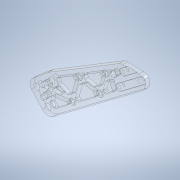
# Autodesk Inventor part: アーム アーム先端根本ポリカパーツ
Saved by Autodesk Inventor 2020.2 (Build 242310000, 310)
## iProperties
Created: 2020-05-02
Part Number: アーム アーム先端根本ポリカパーツ
Material: ポリカーボネート、クリア
Document SubType Name: Modeling
Designer: mozar
Density: 1.2 g/cm^3
Appearance: ポリカーボネート - クリア
Mass: 15.4398 g
Surface Area: 103.612 cm^2
Volume: 12.8665 cm^3
Author: mozar
Autodesk Inventor part; units mm, degrees
(part 1 of 2)
ref_plane "YZ Plane" through (0, 0, 0) normal (1, 0, 0) x (0, 1, 0)
ref_plane "XZ Plane" through (0, 0, 0) normal (0, 1, 0) x (-1, 0, 0)
ref_plane "XY Plane" through (0, 0, 0) normal (0, 0, 1) x (1, 0, 0)
sketch "スケッチ1" plane through (0, 0, 0) normal (0, 0, 1) x (1, 0, 0)
  circle A0 centre (-129.11052, 24.304119) radius 1.5
  circle A1 centre (-99.752673, 43.359743) radius 1.5
  circle A2 centre (-45.703772, 62.415368) radius 1.5
  circle A3 centre (-41.036979, 81.470992) radius 1.5
  circle A4 centre (-70.394826, 62.415368) radius 1.5
  circle A5 centre (-73.694174, 41.402576) radius 1.5
  circle A6 centre (-101.684575, 20.389785) radius 1.5
  circle A7 centre (-147.951739, 7.872185) radius 1.5
  line L0 (-23.449069, 99.142406) -> (-7.448842, 98.649717)
  arc A8 (-3.447491, 86.009971) -> (-7.448842, 98.649717) centre (-7.665058, 91.628045) ccw
  line L1 (-3.447491, 86.009971) -> (-131.660668, -10.24148)
  arc A9 (-141.440781, -10.106867) -> (-131.660668, -10.24148) centre (-136.463592, -3.843674) ccw
  line L2 (-141.440781, -10.106867) -> (-154.18878, 0.023621)
  arc A10 (-153.409815, 16.281111) -> (-154.18878, 0.023621) centre (-147.951739, 7.872185) ccw
  line L3 (-153.409815, 16.281111) -> (-27.490021, 98.013273)
  arc A11 (-23.449069, 99.142406) -> (-27.490021, 98.013273) centre (-23.665285, 92.120734) ccw
  circle A12 centre (-136.463592, -3.843674) radius 1.5
  circle A13 centre (-7.665058, 91.628045) radius 1.5
  circle A14 centre (-27.658202, 76.618908) radius 1.5
  circle A15 centre (-23.665285, 92.120734) radius 1.5
  circle A16 centre (-136.463592, -3.843674) radius 8
  circle A17 centre (-165.894632, -3.310235) radius 1.5
  circle A18 centre (-136.536785, 15.745389) radius 1.5
  circle A19 centre (-82.487883, 34.801014) radius 1.5
  circle A20 centre (-77.821091, 53.856638) radius 1.5
  circle A21 centre (-107.178938, 34.801014) radius 1.5
  circle A22 centre (-110.478285, 13.788222) radius 1.5
  circle A23 centre (-138.468687, -7.22457) radius 1.5
  circle A24 centre (-184.735851, -19.742169) radius 1.5
  circle A25 centre (-173.247704, -31.458028) radius 1.5
  circle A26 centre (-44.44917, 64.013691) radius 1.5
  circle A27 centre (-64.442314, 49.004554) radius 1.5
  circle A28 centre (-60.449397, 64.50638) radius 1.5
  line L4 (-64.274133, 70.398919) -> (-190.193926, -11.333243)
  arc A29 (-190.193926, -11.333243) -> (-190.972891, -27.590733) centre (-184.735851, -19.742169) ccw
  line L5 (-190.972891, -27.590733) -> (-178.224893, -37.721221)
  arc A30 (-178.224893, -37.721221) -> (-168.44478, -37.855834) centre (-173.247704, -31.458028) ccw
  line L6 (-168.44478, -37.855834) -> (-40.231602, 58.395617)
  arc A31 (-40.231602, 58.395617) -> (-44.232954, 71.035362) centre (-44.44917, 64.013691) ccw
  line L7 (-44.232954, 71.035362) -> (-60.233181, 71.528052)
  arc A32 (-60.233181, 71.528052) -> (-64.274133, 70.398919) centre (-60.449397, 64.50638) ccw
  circle A33 centre (-60.449397, 64.50638) radius 7.025
  circle A34 centre (-147.951739, 7.872185) radius 10.025
  line L8 (-153.154364, 16.44151) -> (-64.095126, 70.511318)
  point P0 (0, 0)
  point P1 (0, 0)
  point P2 (36.784112, 27.614354)
  constraints: 35 centre point, 20 point on circle, 18 end point, 2 coincident, 2 tangent, 54 other
extrude "押し出し1" add sketch "スケッチ1" against normal blind 5 contours A0 | A1 | A2 A26 | A4 | A5 | A6 | A34 L4 A10 | L1 A16 A34 L4 A33 L7 A31 | L4 A34 A16 A10 | L8 A32 L4 A34 | A9 A16 A34 | A34 A16 L2 | A32 A33 | A16 A34 | A18 | A19 | A20 | A21 | A22 | A23 picked at (-46.281723, 61.837664)
sketch "スケッチ2" plane through (0, 0, 0) normal (0, 0, 1) x (1, 0, 0)
  circle A0 centre (-64.442314, 49.004554) radius 1.5
  circle A1 centre (-44.44917, 64.013691) radius 1.5
  line L0 (-41.268818, 70.277554) -> (-66.303447, 51.483704)
  arc A2 (-37.546552, 65.319255) -> (-41.268818, 70.277554) centre (-44.44917, 64.013691) ccw
  line L1 (-62.581181, 46.525404) -> (-37.546552, 65.319255)
  arc A3 (-66.303447, 51.483704) -> (-62.581181, 46.525404) centre (-64.442314, 49.004554) ccw
  circle A4 centre (-60.449397, 64.50638) radius 1.5
  line L2 (-46.496021, 71.105048) -> (-56.416161, 71.410515)
  line L3 (-58.588264, 62.02723) -> (-46.496021, 71.105048)
  arc A5 (-62.310529, 66.98553) -> (-58.588264, 62.02723) centre (-60.449397, 64.50638) ccw
  line L4 (-56.416161, 71.410515) -> (-62.310529, 66.98553)
  point P0 (0, 0)
  point P1 (0, 0)
  constraints: 10 end point, 6 centre point, 6 point on circle, 25 other
extrude "押し出し2" cut sketch "スケッチ2" against normal blind 1
sketch "スケッチ3" plane through (0, 0, 0) normal (0, 0, 1) x (1, 0, 0)
  line L0 (-41.268818, 70.277554) -> (-66.303447, 51.483704)
  arc A0 (-66.303447, 51.483704) -> (-62.581181, 46.525404) centre (-64.442314, 49.004554) ccw
  line L1 (-62.581181, 46.525404) -> (-37.546552, 65.319255)
  arc A1 (-40.231602, 58.395617) -> (-37.546552, 65.319255) centre (-44.44917, 64.013691) ccw
  line L2 (-40.231602, 58.395617) -> (-131.660668, -10.24148)
  arc A2 (-141.440781, -10.106867) -> (-131.660668, -10.24148) centre (-136.463592, -3.843674) ccw
  line L3 (-141.440781, -10.106867) -> (-154.18878, 0.023621)
  arc A3 (-153.154364, 16.44151) -> (-154.18878, 0.023621) centre (-147.951739, 7.872185) ccw
  line L4 (-153.154364, 16.44151) -> (-64.095126, 70.511318)
  arc A4 (-60.233181, 71.528052) -> (-64.095126, 70.511318) centre (-60.449397, 64.50638) ccw
  line L5 (-60.233181, 71.528052) -> (-56.416161, 71.410515)
  line L6 (-56.416161, 71.410515) -> (-62.310529, 66.98553)
  arc A5 (-62.310529, 66.98553) -> (-58.588264, 62.02723) centre (-60.449397, 64.50638) ccw
  line L7 (-58.588264, 62.02723) -> (-46.496021, 71.105048)
  line L8 (-46.496021, 71.105048) -> (-44.232954, 71.035362)
  arc A6 (-41.268818, 70.277554) -> (-44.232954, 71.035362) centre (-44.44917, 64.013691) ccw
  circle A7 centre (-136.463592, -3.843674) radius 1.5
  circle A8 centre (-147.951739, 7.872185) radius 1.5
  circle A9 centre (-147.951739, 7.872185) radius 1.5
  circle A10 centre (-147.951739, 7.872185) radius 3
  circle A11 centre (-136.463592, -3.843674) radius 1.5
  circle A12 centre (-136.463592, -3.843674) radius 3
  point P0 (0, 0)
  dimension "d4" = 6
  dimension "d5" = 6
  constraints: 2 centre point, 2 coincident
  measures "d4" diameter of A10
  measures "d5" diameter of A12
extrude "押し出し3" cut sketch "スケッチ3" against normal blind 1 contours A10 | A12
sketch "スケッチ4" plane through (0, 0, 0) normal (0, 0, 1) x (1, 0, 0)
  line L0 (-60.233181, 71.528052) -> (-44.232954, 71.035362)
  arc A0 (-40.231602, 58.395617) -> (-44.232954, 71.035362) centre (-44.44917, 64.013691) ccw
  line L1 (-40.231602, 58.395617) -> (-131.660668, -10.24148)
  arc A1 (-141.440781, -10.106867) -> (-131.660668, -10.24148) centre (-136.463592, -3.843674) ccw
  line L2 (-141.440781, -10.106867) -> (-154.18878, 0.023621)
  arc A2 (-153.154364, 16.44151) -> (-154.18878, 0.023621) centre (-147.951739, 7.872185) ccw
  line L3 (-153.154364, 16.44151) -> (-64.095126, 70.511318)
  arc A3 (-60.233181, 71.528052) -> (-64.095126, 70.511318) centre (-60.449397, 64.50638) ccw
  circle A4 centre (-147.951739, 7.872185) radius 1.5
  circle A5 centre (-136.463592, -3.843674) radius 1.5
  circle A6 centre (-60.449397, 64.50638) radius 1.5
  circle A7 centre (-64.442314, 49.004554) radius 1.5
  circle A8 centre (-44.44917, 64.013691) radius 1.5
  line L4 (-60.721853, 64.955147) -> (-149.781091, 10.885339)
  arc A9 (-149.781091, 10.885339) -> (-150.144813, 5.112465) centre (-147.951739, 7.872185) ccw
  line L5 (-150.144813, 5.112465) -> (-137.396815, -5.018022)
  arc A10 (-137.396815, -5.018022) -> (-135.563044, -5.043262) centre (-136.463592, -3.843674) ccw
  line L6 (-135.563044, -5.043262) -> (-44.133978, 63.593834)
  arc A11 (-44.133978, 63.593834) -> (-44.433011, 64.538442) centre (-44.44917, 64.013691) ccw
  line L7 (-44.433011, 64.538442) -> (-60.433238, 65.031131)
  arc A12 (-60.433238, 65.031131) -> (-60.721853, 64.955147) centre (-60.449397, 64.50638) ccw
  circle A13 centre (-77.811872, 54.579424) radius 3
  circle A14 centre (-84.115857, 33.578871) radius 3
  circle A15 centre (-105.248527, 37.922031) radius 3
  circle A16 centre (-112.106259, 12.566079) radius 3
  circle A17 centre (-132.685182, 21.264639) radius 3
  point P0 (0, 0)
  dimension "d15" = 6.5
  dimension "d16" = 6
  dimension "d17" = 6
  dimension "d18" = 6
  dimension "d19" = 6
  dimension "d20" = 6
  dimension "d21" = 104.18777
  dimension "d22" = 20
  dimension "d25" = 89.33084
  dimension "d26" = 25
  dimension "d27" = 35
  dimension "d28" = 20
  dimension "d29" = 64.19466
  dimension "d30" = 32.09733
  constraints: 9 centre point, 8 end point, 8 point on circle, 5 point on line, 7 other
  measures "d15" distance between parallel lines of L3 L4
  measures "d16" diameter of A13
  measures "d17" diameter of A14
  measures "d18" diameter of A15
  measures "d19" diameter of A16
  measures "d20" diameter of A17
  measures "d21" distance of L4.start L4.end
  measures "d22" distance of A3.centre A13.centre
  measures "d25" distance of A7.centre A5.centre
  measures "d26" distance of A7.centre A14.centre
  measures "d27" distance of A14.centre A16.centre
  measures "d28" distance of L4.end A17.centre
  measures "d29" distance of A13.centre A17.centre
  measures "d30" distance of A13.centre A15.centre
hole "穴2" at (-132.685182, 21.264639, 0) at (-105.248527, 37.922031, 0) at (-77.811872, 54.579424, 0) at (-84.115857, 33.578871, 0) at (-112.106259, 12.566079, 0) direction (0, 0, -1) diameter 3 depth 12 tip angle 118
extrude "押し出し4" cut sketch "スケッチ4" against normal blind 1 contours A16 L6 | L6 A16 | A17 L4 | L4 A17 | A14 L6 | L6 A14 | A15 L4 | L4 A15 | A13 L4 | L4 A13
sketch "スケッチ5" plane through (0, 0, 0) normal (0, 0, 1) x (1, 0, 0)
  circle A0 centre (-132.685182, 21.264639) radius 3
  circle A1 centre (-105.248527, 37.922031) radius 3
  circle A2 centre (-84.115857, 33.578871) radius 3
  circle A3 centre (-77.811872, 54.579424) radius 3
  circle A4 centre (-112.106259, 12.566079) radius 3
  circle A5 centre (-136.463592, -3.843674) radius 3
  circle A6 centre (-147.951739, 7.872185) radius 3
  line L0 (-62.310529, 66.98553) -> (-56.416161, 71.410515)
  line L1 (-56.416161, 71.410515) -> (-60.233181, 71.528052)
  arc A7 (-60.233181, 71.528052) -> (-64.095126, 70.511318) centre (-60.449397, 64.50638) ccw
  line L2 (-64.095126, 70.511318) -> (-153.154364, 16.44151)
  arc A8 (-153.154364, 16.44151) -> (-154.18878, 0.023621) centre (-147.951739, 7.872185) ccw
  line L3 (-154.18878, 0.023621) -> (-141.440781, -10.106867)
  arc A9 (-141.440781, -10.106867) -> (-131.660668, -10.24148) centre (-136.463592, -3.843674) ccw
  line L4 (-131.660668, -10.24148) -> (-40.231602, 58.395617)
  arc A10 (-40.231602, 58.395617) -> (-37.546552, 65.319255) centre (-44.44917, 64.013691) ccw
  line L5 (-37.546552, 65.319255) -> (-62.581181, 46.525404)
  arc A11 (-66.303447, 51.483704) -> (-62.581181, 46.525404) centre (-64.442314, 49.004554) ccw
  line L6 (-66.303447, 51.483704) -> (-41.268818, 70.277554)
  arc A12 (-41.268818, 70.277554) -> (-44.232954, 71.035362) centre (-44.44917, 64.013691) ccw
  line L7 (-44.232954, 71.035362) -> (-46.496021, 71.105048)
  line L8 (-46.496021, 71.105048) -> (-58.588264, 62.02723)
  arc A13 (-62.310529, 66.98553) -> (-58.588264, 62.02723) centre (-60.449397, 64.50638) ccw
  circle A14 centre (-147.951739, 7.872185) radius 1.5
  circle A15 centre (-147.951739, 7.872185) radius 7.5
  circle A16 centre (-136.463592, -3.843674) radius 1.5
  circle A17 centre (-136.463592, -3.843674) radius 7.5
  circle A18 centre (-132.685182, 21.264639) radius 1.5
  circle A19 centre (-132.685182, 21.264639) radius 6.5
  line L9 (-152.614053, 13.746947) -> (-136.725853, 26.3561)
  line L10 (-126.224445, 20.551277) -> (-129.008896, -4.666783)
  line L11 (-153.306826, 2.621181) -> (-141.818679, -9.094678)
  point P0 (0, 0)
  dimension "d40" = 15
  dimension "d42" = 15
  constraints: 7 tangent, 6 end point, 6 point on circle, 3 centre point, 3 coincident
  measures "d40" diameter of A15
  measures "d42" diameter of A17
hole "穴3" at (-147.951739, 7.872185, 0) at (-132.685182, 21.264639, 0) at (-136.463592, -3.843674, 0) direction (0, 0, -1) diameter 6 depth 12 tip angle 118
sketch "スケッチ6" plane through (0, 0, 0) normal (0, 0, 1) x (1, 0, 0)
  circle A0 centre (-132.685182, 21.264639) radius 3
  circle A1 centre (-105.248527, 37.922031) radius 3
  circle A2 centre (-84.115857, 33.578871) radius 3
  circle A3 centre (-77.811872, 54.579424) radius 3
  circle A4 centre (-112.106259, 12.566079) radius 3
  circle A5 centre (-136.463592, -3.843674) radius 3
  circle A6 centre (-147.951739, 7.872185) radius 3
  line L0 (-41.268818, 70.277554) -> (-66.303447, 51.483704)
  arc A7 (-66.303447, 51.483704) -> (-62.581181, 46.525404) centre (-64.442314, 49.004554) ccw
  line L1 (-62.581181, 46.525404) -> (-37.546552, 65.319255)
  arc A8 (-40.231602, 58.395617) -> (-37.546552, 65.319255) centre (-44.44917, 64.013691) ccw
  line L2 (-40.231602, 58.395617) -> (-131.660668, -10.24148)
  arc A9 (-141.440781, -10.106867) -> (-131.660668, -10.24148) centre (-136.463592, -3.843674) ccw
  line L3 (-141.440781, -10.106867) -> (-154.18878, 0.023621)
  arc A10 (-153.154364, 16.44151) -> (-154.18878, 0.023621) centre (-147.951739, 7.872185) ccw
  line L4 (-153.154364, 16.44151) -> (-64.095126, 70.511318)
  arc A11 (-60.233181, 71.528052) -> (-64.095126, 70.511318) centre (-60.449397, 64.50638) ccw
  line L5 (-60.233181, 71.528052) -> (-56.416161, 71.410515)
  line L6 (-56.416161, 71.410515) -> (-62.310529, 66.98553)
  arc A12 (-62.310529, 66.98553) -> (-58.588264, 62.02723) centre (-60.449397, 64.50638) ccw
  line L7 (-58.588264, 62.02723) -> (-46.496021, 71.105048)
  line L8 (-46.496021, 71.105048) -> (-44.232954, 71.035362)
  arc A13 (-41.268818, 70.277554) -> (-44.232954, 71.035362) centre (-44.44917, 64.013691) ccw
  circle A14 centre (-132.685182, 21.264639) radius 8
  circle A15 centre (-147.951739, 7.872185) radius 8
  circle A16 centre (-136.463592, -3.843674) radius 8
  circle A17 centre (-112.106259, 12.566079) radius 8
  circle A18 centre (-105.248527, 37.922031) radius 8
  circle A19 centre (-84.115857, 33.578871) radius 8
  circle A20 centre (-77.811872, 54.579424) radius 8
  point P0 (0, 0)
  dimension "d50" = 5
  dimension "d51" = 5
  dimension "d52" = 5
  dimension "d53" = 5
  dimension "d54" = 5
  dimension "d55" = 5
  dimension "d56" = 5
  constraints: 7 centre point
  measures "d50" radial gap between concentric circles of A0 A14
  measures "d51" radial gap between concentric circles of A6 A15
  measures "d52" radial gap between concentric circles of A5 A16
  measures "d53" radial gap between concentric circles of A4 A17
  measures "d54" radial gap between concentric circles of A1 A18
  measures "d55" radial gap between concentric circles of A2 A19
  measures "d56" radial gap between concentric circles of A3 A20
sketch "スケッチ7" plane through (0, 0, 0) normal (0, 0, 1) x (1, 0, 0)
  circle A0 centre (-132.685182, 21.264639) radius 3
  circle A1 centre (-147.951739, 7.872185) radius 3
  circle A2 centre (-136.463592, -3.843674) radius 3
  circle A3 centre (-84.115857, 33.578871) radius 1.5
  circle A4 centre (-105.248527, 37.922031) radius 1.5
  circle A5 centre (-77.811872, 54.579424) radius 1.5
  circle A6 centre (-112.106259, 12.566079) radius 1.5
  line L0 (-60.233181, 71.528052) -> (-44.232954, 71.035362)
  arc A7 (-40.231602, 58.395617) -> (-44.232954, 71.035362) centre (-44.44917, 64.013691) ccw
  line L1 (-40.231602, 58.395617) -> (-131.660668, -10.24148)
  arc A8 (-141.440781, -10.106867) -> (-131.660668, -10.24148) centre (-136.463592, -3.843674) ccw
  line L2 (-141.440781, -10.106867) -> (-154.18878, 0.023621)
  arc A9 (-153.154364, 16.44151) -> (-154.18878, 0.023621) centre (-147.951739, 7.872185) ccw
  line L3 (-153.154364, 16.44151) -> (-64.095126, 70.511318)
  arc A10 (-60.233181, 71.528052) -> (-64.095126, 70.511318) centre (-60.449397, 64.50638) ccw
  circle A11 centre (-60.449397, 64.50638) radius 1.5
  circle A12 centre (-64.442314, 49.004554) radius 1.5
  circle A13 centre (-44.44917, 64.013691) radius 1.5
  circle A14 centre (-147.951739, 7.872185) radius 6
  circle A15 centre (-132.685182, 21.264639) radius 6
  circle A16 centre (-136.463592, -3.843674) radius 6
  circle A17 centre (-112.106259, 12.566079) radius 1.5
  circle A18 centre (-112.106259, 12.566079) radius 6
  circle A19 centre (-105.248527, 37.922031) radius 1.5
  circle A20 centre (-105.248527, 37.922031) radius 6
  circle A21 centre (-84.115857, 33.578871) radius 1.5
  circle A22 centre (-84.115857, 33.578871) radius 6
  circle A23 centre (-77.811872, 54.579424) radius 1.5
  circle A24 centre (-77.811872, 54.579424) radius 6
  circle A25 centre (-64.442314, 49.004554) radius 1.5
  line L4 (-56.416161, 71.410515) -> (-46.496021, 71.105048)
  line L5 (-62.310529, 66.98553) -> (-56.416161, 71.410515)
  arc A26 (-62.310529, 66.98553) -> (-58.588264, 62.02723) centre (-60.449397, 64.50638) ccw
  line L6 (-46.496021, 71.105048) -> (-58.588264, 62.02723)
  circle A27 centre (-60.449397, 64.50638) radius 1.5
  arc A28 (-66.303447, 51.483704) -> (-62.581181, 46.525404) centre (-64.442314, 49.004554) ccw
  line L7 (-37.546552, 65.319255) -> (-62.581181, 46.525404)
  arc A29 (-37.546552, 65.319255) -> (-41.268818, 70.277554) centre (-44.44917, 64.013691) ccw
  line L8 (-66.303447, 51.483704) -> (-41.268818, 70.277554)
  circle A30 centre (-64.442314, 49.004554) radius 1.5
  circle A31 centre (-44.44917, 64.013691) radius 1.5
  arc A32 (-65.312357, 70.984158) -> (-55.586436, 58.028601) centre (-60.449397, 64.50638) ccw
  line L9 (-65.312357, 70.984158) -> (-58.015345, 76.462128)
  line L10 (-58.015345, 76.462128) -> (-32.094978, 75.663972)
  line L11 (-32.094978, 75.663972) -> (-55.586436, 58.028601)
  arc A33 (-69.305274, 55.482332) -> (-59.579353, 42.526775) centre (-64.442314, 49.004554) ccw
  line L12 (-69.305274, 55.482332) -> (-42.204434, 75.827318)
  arc A34 (-32.478513, 62.87176) -> (-42.204434, 75.827318) centre (-44.44917, 64.013691) ccw
  line L13 (-32.478513, 62.87176) -> (-59.579353, 42.526775)
  line L14 (-61.500301, 66.237341) -> (-150.559539, 12.167532)
  arc A35 (-150.559539, 12.167532) -> (-151.078036, 3.938117) centre (-147.951739, 7.872185) ccw
  line L15 (-151.078036, 3.938117) -> (-138.330038, -6.192371)
  arc A36 (-138.330038, -6.192371) -> (-134.662496, -6.242851) centre (-136.463592, -3.843674) ccw
  line L16 (-134.662496, -6.242851) -> (-43.23343, 62.394246)
  arc A37 (-43.23343, 62.394246) -> (-44.386844, 66.037731) centre (-44.44917, 64.013691) ccw
  line L17 (-44.386844, 66.037731) -> (-60.387071, 66.53042)
  arc A38 (-60.387071, 66.53042) -> (-61.500301, 66.237341) centre (-60.449397, 64.50638) ccw
  line L18 (-136.463592, -3.843674) -> (-132.685182, 21.264639) construction
  line L19 (-134.48586, -4.141291) -> (-130.70745, 20.967021)
  line L20 (-134.662913, 21.562257) -> (-138.441324, -3.546056)
  arc A39 (-138.441324, -3.546056) -> (-134.48586, -4.141291) centre (-136.463592, -3.843674) ccw
  arc A40 (-130.70745, 20.967021) -> (-134.662913, 21.562257) centre (-132.685182, 21.264639) ccw
  circle A41 centre (-132.685182, 21.264639) radius 3
  circle A42 centre (-112.106259, 12.566079) radius 3
  line L21 (-132.685182, 21.264639) -> (-112.106259, 12.566079) construction
  line L22 (-133.463861, 19.422451) -> (-112.884938, 10.723891)
  line L23 (-111.327579, 14.408267) -> (-131.906502, 23.106828)
  arc A43 (-131.906502, 23.106828) -> (-133.463861, 19.422451) centre (-132.685182, 21.264639) ccw
  arc A44 (-112.884938, 10.723891) -> (-111.327579, 14.408267) centre (-112.106259, 12.566079) ccw
  line L24 (-112.106259, 12.566079) -> (-105.248527, 37.922031) construction
  line L25 (-110.175624, 12.043922) -> (-103.317891, 37.399875)
  line L26 (-107.179162, 38.444188) -> (-114.036894, 13.088236)
  arc A45 (-114.036894, 13.088236) -> (-110.175624, 12.043922) centre (-112.106259, 12.566079) ccw
  arc A46 (-103.317891, 37.399875) -> (-107.179162, 38.444188) centre (-105.248527, 37.922031) ccw
  line L27 (-105.248527, 37.922031) -> (-84.115857, 33.578871) construction
  line L28 (-105.651149, 35.962977) -> (-84.51848, 31.619816)
  line L29 (-83.713234, 35.537925) -> (-104.845904, 39.881086)
  arc A47 (-104.845904, 39.881086) -> (-105.651149, 35.962977) centre (-105.248527, 37.922031) ccw
  arc A48 (-84.51848, 31.619816) -> (-83.713234, 35.537925) centre (-84.115857, 33.578871) ccw
  line L30 (-84.115857, 33.578871) -> (-77.811872, 54.579424) construction
  line L31 (-82.2003, 33.003855) -> (-75.896315, 54.004408)
  line L32 (-79.727428, 55.154439) -> (-86.031414, 34.153886)
  arc A49 (-86.031414, 34.153886) -> (-82.2003, 33.003855) centre (-84.115857, 33.578871) ccw
  arc A50 (-75.896315, 54.004408) -> (-79.727428, 55.154439) centre (-77.811872, 54.579424) ccw
  circle A51 centre (-144.704037, -0.330722) radius 1
  line L33 (-77.811872, 54.579424) -> (-64.442314, 49.004554) construction
  line L34 (-78.581599, 52.733477) -> (-65.212041, 47.158607)
  line L35 (-63.672586, 50.850501) -> (-77.042144, 56.425371)
  arc A52 (-77.042144, 56.425371) -> (-78.581599, 52.733477) centre (-77.811872, 54.579424) ccw
  arc A53 (-65.212041, 47.158607) -> (-63.672586, 50.850501) centre (-64.442314, 49.004554) ccw
  point P0 (0, 0)
  point P1 (-134.574387, 8.710483)
  point P2 (-122.39572, 16.915359)
  point P3 (-108.677393, 25.244055)
  point P4 (-94.682192, 35.750451)
  point P5 (-80.963864, 44.079147)
  point P6 (-68.204283, 62.167206)
  point P7 (-73.624406, 58.876531)
  point P8 (-69.826103, 55.056397)
  point P9 (-65.605749, 58.259618)
  point P10 (-77.522704, 48.586396)
  point P11 (-80.573911, 38.421868)
  point P12 (-78.569322, 35.86709)
  point P13 (-69.498656, 42.676568)
  point P14 (-72.530668, 48.570357)
  point P15 (-84.405025, 39.571898)
  point P16 (-81.353818, 49.736427)
  point P17 (-83.556232, 52.846703)
  point P18 (-101.061061, 42.219139)
  point P19 (-99.304861, 38.742298)
  point P20 (-89.254278, 36.676714)
  point P21 (-90.059523, 32.758605)
  point P22 (-100.110106, 34.824188)
  point P23 (-104.794773, 31.939214)
  point P24 (-108.698741, 17.504583)
  point P25 (-106.559724, 14.854299)
  point P26 (-87.861296, 28.891474)
  point P27 (-112.560012, 18.548897)
  point P28 (-108.656044, 32.983527)
  point P29 (-110.992887, 36.18931)
  point P30 (-128.497716, 25.561747)
  point P31 (-126.696006, 20.904389)
  point P32 (-116.538075, 16.610706)
  point P33 (-118.095434, 12.926329)
  point P34 (-128.253365, 17.220012)
  point P35 (-131.54924, 15.373151)
  point P36 (-133.64407, 1.452579)
  point P37 (-130.506999, -3.12326)
  point P38 (-115.851697, 7.878682)
  point P39 (-137.599533, 2.047815)
  point P40 (-135.504704, 15.968386)
  point P41 (-138.429542, 19.531918)
  point P42 (-147.756986, 13.869023)
  point P43 (-71.127093, 51.791989)
  point P44 (-36.093963, 72.661877)
  point P45 (-44.896836, 66.053435)
  point P46 (-54.816977, 66.358902)
  point P47 (-79.721107, 55.175091)
  point P48 (-77.459531, 56.548143)
  point P49 (-71.821018, 54.248253)
  point P50 (-70.917193, 53.871374)
  point P51 (-72.456648, 50.17948)
  point P52 (-73.360473, 50.556359)
  point P53 (-142.398101, -2.959592)
  point P54 (-148.511205, 1.898325)
  dimension "d57" = 3
  dimension "d58" = 3
  dimension "d59" = 3
  dimension "d60" = 12
  dimension "d61" = 12
  dimension "d62" = 12
  dimension "d63" = 12
  dimension "d65" = 5
  dimension "d66" = 5
  dimension "d67" = 5
  dimension "d68" = 4
  dimension "d69" = 4
  dimension "d70" = 4
  dimension "d71" = 4
  dimension "d72" = 4
  dimension "d73" = 2
  dimension "d77" = 4
  constraints: 66 end point, 38 point on circle, 27 centre point, 24 tangent, 6 midpoint, 6 parallel, 4 coincident, 13 other
  measures "d57" radial gap between concentric circles of A1 A14
  measures "d58" radial gap between concentric circles of A0 A15
  measures "d59" radial gap between concentric circles of A2 A16
  measures "d60" diameter of A18
  measures "d61" diameter of A20
  measures "d62" diameter of A22
  measures "d63" diameter of A24
  measures "d65" radial gap between concentric circles of A26 A32
  measures "d66" distance between parallel lines of L7 L13
  measures "d67" distance between parallel lines of L3 L14
  measures "d68" diameter of A40
  measures "d69" diameter of A44
  measures "d70" diameter of A46
  measures "d71" diameter of A48
  measures "d72" diameter of A50
  measures "d73" diameter of A51
  measures "d77" diameter of A53
extrude "押し出し6" cut sketch "スケッチ7" against normal blind 4 contours A15 L14 A20 L26 A18 L23 | L22 A18 L16 A16 L19 A15 | A15 L20 A16 L15 A51 A14 L14 | L14 A24 L32 A22 L29 A20 | L25 A20 L28 A22 L16 A18 | A51 L15 | L14 A32 L12 A33 L35 A24 | A24 L34 A33 L16 A22 L31 picked at (-144.701859, -0.863759)
fillet "フィレット1" radius 1 41 edges at (-65.6057, 58.2596, -2) (-68.2043, 62.1672, -2) (-73.6244, 58.8765, -2) (-71.821, 54.2483, -2) (-70.9172, 53.8714, -2) (-73.3605, 50.5564, -2) (-72.4566, 50.1795, -2) (-77.5227, 48.5864, -2) (-69.4987, 42.6766, -2) (-78.5693, 35.8671, -2) (-80.5739, 38.4219, -2) (-84.405, 39.5719, -2) (-81.3538, 49.7364, -2) (-83.5562, 52.8467, -2) (-101.0611, 42.2191, -2) (-99.3049, 38.7423, -2) (-89.2543, 36.6767, -2) (-90.0595, 32.7586, -2) (-87.8613, 28.8915, -2) (-100.1101, 34.8242, -2) (-104.7948, 31.9392, -2) (-108.6987, 17.5046, -2) (-106.5597, 14.8543, -2) (-112.56, 18.5489, -2) (-116.5381, 16.6107, -2) (-108.656, 32.9835, -2) (-110.9929, 36.1893, -2) (-126.696, 20.9044, -2) (-128.4977, 25.5617, -2) (-128.2534, 17.22, -2) (-131.5492, 15.3732, -2) (-118.0954, 12.9263, -2) (-115.8517, 7.8787, -2) (-130.507, -3.1233, -2) (-133.6441, 1.4526, -2) (-137.5995, 2.0478, -2) (-142.3981, -2.9596, -2) (-135.5047, 15.9684, -2) (-138.4295, 19.5319, -2) (-147.757, 13.869, -2) (-148.5112, 1.8983, -2)
sketch "スケッチ8" plane through (0, 0, 0) normal (0, 0, 1) x (1, 0, 0)
  arc A0 (-110.586613, 35.182536) -> (-109.14609, 33.360343) centre (-105.248527, 37.922031) ccw
  arc A1 (-108.830366, 32.338983) -> (-109.14609, 33.360343) centre (-109.795684, 32.600062) ccw
  line L0 (-108.830366, 32.338983) -> (-112.38569, 19.19344)
  arc A2 (-113.173186, 18.470456) -> (-112.38569, 19.19344) centre (-113.351007, 19.454519) ccw
  arc A3 (-113.173186, 18.470456) -> (-116.098395, 17.045236) centre (-112.106259, 12.566079) ccw
  arc A4 (-117.15309, 16.870668) -> (-116.098395, 17.045236) centre (-116.763751, 17.791763) ccw
  line L1 (-117.15309, 16.870668) -> (-126.080991, 20.644427)
  arc A5 (-126.690727, 21.522538) -> (-126.080991, 20.644427) centre (-125.691651, 21.565521) ccw
  arc A6 (-126.690727, 21.522538) -> (-127.791923, 24.736817) centre (-132.685182, 21.264639) ccw
  arc A7 (-127.495344, 26.170308) -> (-127.791923, 24.736817) centre (-126.976379, 25.315513) ccw
  line L2 (-127.495344, 26.170308) -> (-111.995259, 35.580749)
  arc A8 (-110.586613, 35.182536) -> (-111.995259, 35.580749) centre (-111.476294, 34.725953) ccw
  arc A9 (-71.858452, 55.325612) -> (-70.160292, 54.741689) centre (-70.866216, 55.449977) ccw
  arc A10 (-71.858452, 55.325612) -> (-72.918613, 58.051601) centre (-77.811872, 54.579424) ccw
  arc A11 (-72.622035, 59.485093) -> (-72.918613, 58.051601) centre (-72.10307, 58.630298) ccw
  line L3 (-72.622035, 59.485093) -> (-69.229438, 61.544813)
  arc A12 (-67.802662, 61.109398) -> (-69.229438, 61.544813) centre (-68.710473, 60.690017) ccw
  arc A13 (-67.802662, 61.109398) -> (-66.414464, 59.026602) centre (-60.449397, 64.50638) ccw
  arc A14 (-66.550527, 57.55036) -> (-66.414464, 59.026602) centre (-67.150892, 58.350086) ccw
  line L4 (-66.550527, 57.55036) -> (-69.305274, 55.482332)
  arc A15 (-69.305274, 55.482332) -> (-70.160292, 54.741689) centre (-64.442314, 49.004554) ccw
  arc A16 (-72.542276, 49.029257) -> (-70.331118, 43.4429) centre (-64.442314, 49.004554) ccw
  arc A17 (-70.457765, 41.956551) -> (-70.331118, 43.4429) centre (-71.058131, 42.756277) ccw
  line L5 (-70.457765, 41.956551) -> (-77.631528, 36.571106)
  arc A18 (-79.072459, 36.829123) -> (-77.631528, 36.571106) centre (-78.231893, 37.370832) ccw
  arc A19 (-79.072459, 36.829123) -> (-80.094406, 38.031727) centre (-84.115857, 33.578871) ccw
  arc A20 (-80.381942, 39.061377) -> (-80.094406, 38.031727) centre (-79.424164, 38.77387) ccw
  line L6 (-80.381942, 39.061377) -> (-77.714673, 47.946886)
  arc A21 (-76.907606, 48.647957) -> (-77.714673, 47.946886) centre (-76.756895, 47.659379) ccw
  arc A22 (-76.907606, 48.647957) -> (-74.152214, 49.824752) centre (-77.811872, 54.579424) ccw
  arc A23 (-72.542276, 49.029257) -> (-74.152214, 49.824752) centre (-73.542271, 49.032306) ccw
  line L7 (-127.63835, 16.96005) -> (-118.71045, 13.186292)
  arc A24 (-118.100714, 12.30818) -> (-118.71045, 13.186292) centre (-119.099789, 12.265197) ccw
  arc A25 (-118.100714, 12.30818) -> (-116.635058, 8.630348) centre (-112.106259, 12.566079) ccw
  arc A26 (-116.789492, 7.174667) -> (-116.635058, 8.630348) centre (-117.389857, 7.974392) ccw
  line L8 (-116.789492, 7.174667) -> (-129.297772, -2.215477)
  arc A27 (-130.83606, -1.762597) -> (-129.297772, -2.215477) centre (-129.898137, -1.415751) ccw
  arc A28 (-130.83606, -1.762597) -> (-133.114093, 1.134364) centre (-136.463592, -3.843674) ccw
  arc A29 (-133.54471, 2.112846) -> (-133.114093, 1.134364) centre (-132.555844, 1.964037) ccw
  line L9 (-133.54471, 2.112846) -> (-131.6486, 14.712884)
  arc A30 (-130.949084, 15.521298) -> (-131.6486, 14.712884) centre (-130.659734, 14.564075) ccw
  arc A31 (-130.949084, 15.521298) -> (-128.693046, 16.785482) centre (-132.685182, 21.264639) ccw
  arc A32 (-127.63835, 16.96005) -> (-128.693046, 16.785482) centre (-128.02769, 16.038956) ccw
  line L10 (-99.456074, 34.689773) -> (-90.713554, 32.89302)
  arc A33 (-89.943579, 32.151404) -> (-90.713554, 32.89302) centre (-90.914866, 31.913493) ccw
  arc A34 (-89.943579, 32.151404) -> (-88.644656, 29.643139) centre (-84.115857, 33.578871) ccw
  arc A35 (-88.79909, 28.187458) -> (-88.644656, 29.643139) centre (-89.399456, 28.987184) ccw
  line L11 (-88.79909, 28.187458) -> (-105.621929, 15.558314)
  arc A36 (-107.062861, 15.816331) -> (-105.621929, 15.558314) centre (-106.222295, 16.35804) ccw
  arc A37 (-107.062861, 15.816331) -> (-108.208695, 17.127767) centre (-112.106259, 12.566079) ccw
  arc A38 (-108.524419, 18.149127) -> (-108.208695, 17.127767) centre (-107.559102, 17.888049) ccw
  line L12 (-108.524419, 18.149127) -> (-104.969096, 31.29467)
  arc A39 (-104.181599, 32.017655) -> (-104.969096, 31.29467) centre (-104.003778, 31.033592) ccw
  arc A40 (-104.181599, 32.017655) -> (-100.45612, 34.311929) centre (-105.248527, 37.922031) ccw
  arc A41 (-99.456074, 34.689773) -> (-100.45612, 34.311929) centre (-99.657386, 33.710245) ccw
  line L13 (-100.058689, 42.827701) -> (-84.558604, 52.238141)
  arc A42 (-83.149958, 51.839928) -> (-84.558604, 52.238141) centre (-84.039639, 51.383346) ccw
  arc A43 (-83.149958, 51.839928) -> (-81.833323, 50.126568) centre (-77.811872, 54.579424) ccw
  arc A44 (-81.545787, 49.096917) -> (-81.833323, 50.126568) centre (-82.503565, 49.384425) ccw
  line L14 (-81.545787, 49.096917) -> (-84.213055, 40.211408)
  arc A45 (-85.020123, 39.510338) -> (-84.213055, 40.211408) centre (-85.170834, 40.498916) ccw
  arc A46 (-85.020123, 39.510338) -> (-88.908264, 37.188973) centre (-84.115857, 33.578871) ccw
  arc A47 (-89.908309, 36.81113) -> (-88.908264, 37.188973) centre (-89.706998, 37.790657) ccw
  line L15 (-89.908309, 36.81113) -> (-98.650829, 38.607882)
  arc A48 (-99.420805, 39.349498) -> (-98.650829, 38.607882) centre (-98.449518, 39.587409) ccw
  arc A49 (-99.420805, 39.349498) -> (-100.355268, 41.394209) centre (-105.248527, 37.922031) ccw
  arc A50 (-100.058689, 42.827701) -> (-100.355268, 41.394209) centre (-99.539724, 41.972905) ccw
  line L16 (-143.581885, -2.018871) -> (-146.594315, 0.375026)
  arc A51 (-146.254963, 2.117105) -> (-146.594315, 0.375026) centre (-145.972167, 1.157925) ccw
  arc A52 (-146.254963, 2.117105) -> (-145.546046, 13.368787) centre (-147.951739, 7.872185) ccw
  arc A53 (-145.664062, 15.139683) -> (-145.546046, 13.368787) centre (-145.145097, 14.284888) ccw
  line L17 (-145.664062, 15.139683) -> (-139.431914, 18.923356)
  arc A54 (-138.023268, 18.525143) -> (-139.431914, 18.923356) centre (-138.912949, 18.068561) ccw
  arc A55 (-138.023268, 18.525143) -> (-136.03468, 16.286601) centre (-132.685182, 21.264639) ccw
  arc A56 (-135.604064, 15.308119) -> (-136.03468, 16.286601) centre (-136.59293, 15.456928) ccw
  line L18 (-135.604064, 15.308119) -> (-137.500173, 2.708082)
  arc A57 (-138.19969, 1.899667) -> (-137.500173, 2.708082) centre (-138.489039, 2.856891) ccw
  arc A58 (-138.19969, 1.899667) -> (-142.031716, -1.608501) centre (-136.463592, -3.843674) ccw
  arc A59 (-143.581885, -2.018871) -> (-142.031716, -1.608501) centre (-142.959736, -1.235972) ccw
  circle A60 centre (-132.685182, 21.264639) radius 3
  circle A61 centre (-105.248527, 37.922031) radius 3
  circle A62 centre (-84.115857, 33.578871) radius 3
  circle A63 centre (-77.811872, 54.579424) radius 3
  circle A64 centre (-112.106259, 12.566079) radius 3
  circle A65 centre (-136.463592, -3.843674) radius 3
  circle A66 centre (-147.951739, 7.872185) radius 3
  line L19 (-62.310529, 66.98553) -> (-56.416161, 71.410515)
  line L20 (-56.416161, 71.410515) -> (-60.233181, 71.528052)
  arc A67 (-60.233181, 71.528052) -> (-64.095126, 70.511318) centre (-60.449397, 64.50638) ccw
  line L21 (-64.095126, 70.511318) -> (-153.154364, 16.44151)
  arc A68 (-153.154364, 16.44151) -> (-154.18878, 0.023621) centre (-147.951739, 7.872185) ccw
  line L22 (-154.18878, 0.023621) -> (-141.440781, -10.106867)
  arc A69 (-141.440781, -10.106867) -> (-131.660668, -10.24148) centre (-136.463592, -3.843674) ccw
  line L23 (-131.660668, -10.24148) -> (-40.231602, 58.395617)
  arc A70 (-40.231602, 58.395617) -> (-37.546552, 65.319255) centre (-44.44917, 64.013691) ccw
  line L24 (-37.546552, 65.319255) -> (-62.581181, 46.525404)
  arc A71 (-66.303447, 51.483704) -> (-62.581181, 46.525404) centre (-64.442314, 49.004554) ccw
  line L25 (-66.303447, 51.483704) -> (-41.268818, 70.277554)
  arc A72 (-41.268818, 70.277554) -> (-44.232954, 71.035362) centre (-44.44917, 64.013691) ccw
  line L26 (-44.232954, 71.035362) -> (-46.496021, 71.105048)
  line L27 (-46.496021, 71.105048) -> (-58.588264, 62.02723)
  arc A73 (-62.310529, 66.98553) -> (-58.588264, 62.02723) centre (-60.449397, 64.50638) ccw
  line L28 (-147.951739, 7.872185) -> (-112.106259, 12.566079) construction
  line L29 (-147.69206, 5.889115) -> (-111.84658, 10.583009)
  line L30 (-112.365938, 14.549149) -> (-148.211419, 9.855255)
  arc A74 (-148.211419, 9.855255) -> (-147.69206, 5.889115) centre (-147.951739, 7.872185) ccw
  arc A75 (-111.84658, 10.583009) -> (-112.365938, 14.549149) centre (-112.106259, 12.566079) ccw
  point P0 (0, 0)
  point P1 (-130.028999, 10.219132)
  point P2 (-119.671463, 13.592505)
  point P3 (-132.06135, 11.970074)
  point P4 (-132.68063, 7.854832)
  point P5 (-117.455549, 9.848526)
  point P6 (-136.1877, 11.429737)
  point P7 (-142.602449, 10.589738)
  point P8 (-142.083091, 6.623598)
  point P9 (-136.80698, 7.314494)
  dimension "d81" = 4
  constraints: 8 end point, 4 point on circle, 4 tangent, 2 centre point, 1 midpoint, 1 parallel
  measures "d81" diameter of A75
extrude "押し出し7" add sketch "スケッチ8" against normal blind 5 contours L7 A24 A25 L29 L9 L30 | L18 L29 A52 L30
fillet "フィレット2" radius 1 8 edges at (-142.0831, 6.6236, -2) (-136.807, 7.3145, -2) (-132.6806, 7.8548, -2) (-132.0614, 11.9701, -2) (-136.1877, 11.4297, -2) (-142.6024, 10.5897, -2) (-119.6715, 13.5925, -2) (-117.4555, 9.8485, -2)
sketch "スケッチ9" plane through (0, 0, -5) normal (0, 0, -1) x (-1, 0, 0)
  arc A0 (116.635058, 8.630348) -> (117.147544, 9.312551) centre (112.106259, 12.566079) ccw
  arc A1 (116.635058, 8.630348) -> (116.789492, 7.174667) centre (117.389857, 7.974392) ccw
  line L0 (116.789492, 7.174667) -> (129.297772, -2.215477)
  arc A2 (129.297772, -2.215477) -> (130.83606, -1.762597) centre (129.898137, -1.415751) ccw
  arc A3 (133.114093, 1.134364) -> (130.83606, -1.762597) centre (136.463592, -3.843674) ccw
  arc A4 (133.114093, 1.134364) -> (133.54471, 2.112846) centre (132.555844, 1.964037) ccw
  line L1 (133.54471, 2.112846) -> (132.792729, 7.109914)
  arc A5 (132.792729, 7.109914) -> (131.933702, 7.95264) centre (131.803863, 6.961105) ccw
  line L2 (131.933702, 7.95264) -> (118.117598, 9.761832)
  arc A6 (118.117598, 9.761832) -> (117.147544, 9.312551) centre (117.987758, 8.770297) ccw
  arc A7 (145.546046, 13.368787) -> (142.910454, 11.125713) centre (147.951739, 7.872185) ccw
  arc A8 (145.546046, 13.368787) -> (145.664062, 15.139683) centre (145.145097, 14.284888) ccw
  line L3 (145.664062, 15.139683) -> (139.431914, 18.923356)
  arc A9 (139.431914, 18.923356) -> (138.023268, 18.525143) centre (138.912949, 18.068561) ccw
  arc A10 (136.03468, 16.286601) -> (138.023268, 18.525143) centre (132.685182, 21.264639) ccw
  arc A11 (136.03468, 16.286601) -> (135.604064, 15.308119) centre (136.59293, 15.456928) ccw
  line L4 (135.604064, 15.308119) -> (136.075602, 12.174654)
  arc A12 (136.075602, 12.174654) -> (136.934628, 11.331928) centre (137.064468, 12.323463) ccw
  line L5 (136.934628, 11.331928) -> (141.9404, 10.676432)
  arc A13 (141.9404, 10.676432) -> (142.910454, 11.125713) centre (142.07024, 11.667967) ccw
  arc A14 (109.14609, 33.360343) -> (110.586613, 35.182536) centre (105.248527, 37.922031) ccw
  arc A15 (109.14609, 33.360343) -> (108.830366, 32.338983) centre (109.795684, 32.600062) ccw
  line L6 (108.830366, 32.338983) -> (112.38569, 19.19344)
  arc A16 (112.38569, 19.19344) -> (113.173186, 18.470456) centre (113.351007, 19.454519) ccw
  arc A17 (116.098395, 17.045236) -> (113.173186, 18.470456) centre (112.106259, 12.566079) ccw
  arc A18 (116.098395, 17.045236) -> (117.15309, 16.870668) centre (116.763751, 17.791763) ccw
  line L7 (117.15309, 16.870668) -> (126.080991, 20.644427)
  arc A19 (126.080991, 20.644427) -> (126.690727, 21.522538) centre (125.691651, 21.565521) ccw
  arc A20 (127.791923, 24.736817) -> (126.690727, 21.522538) centre (132.685182, 21.264639) ccw
  arc A21 (127.791923, 24.736817) -> (127.495344, 26.170308) centre (126.976379, 25.315513) ccw
  line L8 (127.495344, 26.170308) -> (111.995259, 35.580749)
  arc A22 (111.995259, 35.580749) -> (110.586613, 35.182536) centre (111.476294, 34.725953) ccw
  arc A23 (70.160292, 54.741689) -> (71.858452, 55.325612) centre (70.866216, 55.449977) ccw
  arc A24 (72.918613, 58.051601) -> (71.858452, 55.325612) centre (77.811872, 54.579424) ccw
  arc A25 (72.918613, 58.051601) -> (72.622035, 59.485093) centre (72.10307, 58.630298) ccw
  line L9 (72.622035, 59.485093) -> (69.229438, 61.544813)
  arc A26 (69.229438, 61.544813) -> (67.802662, 61.109398) centre (68.710473, 60.690017) ccw
  arc A27 (66.414464, 59.026602) -> (67.802662, 61.109398) centre (60.449397, 64.50638) ccw
  arc A28 (66.414464, 59.026602) -> (66.550527, 57.55036) centre (67.150892, 58.350086) ccw
  line L10 (66.550527, 57.55036) -> (69.305274, 55.482332)
  arc A29 (70.160292, 54.741689) -> (69.305274, 55.482332) centre (64.442314, 49.004554) ccw
  arc A30 (70.331118, 43.4429) -> (72.542276, 49.029257) centre (64.442314, 49.004554) ccw
  arc A31 (70.331118, 43.4429) -> (70.457765, 41.956551) centre (71.058131, 42.756277) ccw
  line L11 (70.457765, 41.956551) -> (77.631528, 36.571106)
  arc A32 (77.631528, 36.571106) -> (79.072459, 36.829123) centre (78.231893, 37.370832) ccw
  arc A33 (80.094406, 38.031727) -> (79.072459, 36.829123) centre (84.115857, 33.578871) ccw
  arc A34 (80.094406, 38.031727) -> (80.381942, 39.061377) centre (79.424164, 38.77387) ccw
  line L12 (80.381942, 39.061377) -> (77.714673, 47.946886)
  arc A35 (77.714673, 47.946886) -> (76.907606, 48.647957) centre (76.756895, 47.659379) ccw
  arc A36 (74.152214, 49.824752) -> (76.907606, 48.647957) centre (77.811872, 54.579424) ccw
  arc A37 (74.152214, 49.824752) -> (72.542276, 49.029257) centre (73.542271, 49.032306) ccw
  line L13 (123.324226, 13.114183) -> (130.745103, 12.142434)
  arc A38 (130.745103, 12.142434) -> (131.863809, 13.282778) centre (130.874943, 13.133969) ccw
  line L14 (131.863809, 13.282778) -> (131.6486, 14.712884)
  arc A39 (131.6486, 14.712884) -> (130.949084, 15.521298) centre (130.659734, 14.564075) ccw
  arc A40 (128.693046, 16.785482) -> (130.949084, 15.521298) centre (132.685182, 21.264639) ccw
  arc A41 (128.693046, 16.785482) -> (127.63835, 16.96005) centre (128.02769, 16.038956) ccw
  line L15 (127.63835, 16.96005) -> (123.064726, 15.026812)
  arc A42 (123.064726, 15.026812) -> (123.324226, 13.114183) centre (123.454066, 14.105718) ccw
  line L16 (99.456074, 34.689773) -> (90.713554, 32.89302)
  arc A43 (90.713554, 32.89302) -> (89.943579, 32.151404) centre (90.914866, 31.913493) ccw
  arc A44 (88.644656, 29.643139) -> (89.943579, 32.151404) centre (84.115857, 33.578871) ccw
  arc A45 (88.644656, 29.643139) -> (88.79909, 28.187458) centre (89.399456, 28.987184) ccw
  line L17 (88.79909, 28.187458) -> (105.621929, 15.558314)
  arc A46 (105.621929, 15.558314) -> (107.062861, 15.816331) centre (106.222295, 16.35804) ccw
  arc A47 (108.208695, 17.127767) -> (107.062861, 15.816331) centre (112.106259, 12.566079) ccw
  arc A48 (108.208695, 17.127767) -> (108.524419, 18.149127) centre (107.559102, 17.888049) ccw
  line L18 (108.524419, 18.149127) -> (104.969096, 31.29467)
  arc A49 (104.969096, 31.29467) -> (104.181599, 32.017655) centre (104.003778, 31.033592) ccw
  arc A50 (100.45612, 34.311929) -> (104.181599, 32.017655) centre (105.248527, 37.922031) ccw
  arc A51 (100.45612, 34.311929) -> (99.456074, 34.689773) centre (99.657386, 33.710245) ccw
  line L19 (100.058689, 42.827701) -> (84.558604, 52.238141)
  arc A52 (84.558604, 52.238141) -> (83.149958, 51.839928) centre (84.039639, 51.383346) ccw
  arc A53 (81.833323, 50.126568) -> (83.149958, 51.839928) centre (77.811872, 54.579424) ccw
  arc A54 (81.833323, 50.126568) -> (81.545787, 49.096917) centre (82.503565, 49.384425) ccw
  line L20 (81.545787, 49.096917) -> (84.213055, 40.211408)
  arc A55 (84.213055, 40.211408) -> (85.020123, 39.510338) centre (85.170834, 40.498916) ccw
  arc A56 (88.908264, 37.188973) -> (85.020123, 39.510338) centre (84.115857, 33.578871) ccw
  arc A57 (88.908264, 37.188973) -> (89.908309, 36.81113) centre (89.706998, 37.790657) ccw
  line L21 (89.908309, 36.81113) -> (98.650829, 38.607882)
  arc A58 (98.650829, 38.607882) -> (99.420805, 39.349498) centre (98.449518, 39.587409) ccw
  arc A59 (100.355268, 41.394209) -> (99.420805, 39.349498) centre (105.248527, 37.922031) ccw
  arc A60 (100.355268, 41.394209) -> (100.058689, 42.827701) centre (99.539724, 41.972905) ccw
  line L22 (141.421042, 6.710292) -> (138.123227, 7.142135)
  arc A61 (138.123227, 7.142135) -> (137.004522, 6.001791) centre (137.993388, 6.1506) ccw
  line L23 (137.004522, 6.001791) -> (137.500173, 2.708082)
  arc A62 (137.500173, 2.708082) -> (138.19969, 1.899667) centre (138.489039, 2.856891) ccw
  arc A63 (142.031716, -1.608501) -> (138.19969, 1.899667) centre (136.463592, -3.843674) ccw
  arc A64 (142.031716, -1.608501) -> (143.581885, -2.018871) centre (142.959736, -1.235972) ccw
  line L24 (143.581885, -2.018871) -> (146.594315, 0.375026)
  arc A65 (146.594315, 0.375026) -> (146.254963, 2.117105) centre (145.972167, 1.157925) ccw
  arc A66 (142.242708, 6.02639) -> (146.254963, 2.117105) centre (147.951739, 7.872185) ccw
  arc A67 (142.242708, 6.02639) -> (141.421042, 6.710292) centre (141.291203, 5.718757) ccw
  circle A68 centre (132.685182, 21.264639) radius 3
  circle A69 centre (105.248527, 37.922031) radius 3
  circle A70 centre (84.115857, 33.578871) radius 3
  circle A71 centre (77.811872, 54.579424) radius 3
  circle A72 centre (112.106259, 12.566079) radius 3
  circle A73 centre (136.463592, -3.843674) radius 3
  circle A74 centre (147.951739, 7.872185) radius 3
  line L25 (62.310529, 66.98553) -> (56.416161, 71.410515)
  line L26 (56.416161, 71.410515) -> (60.233181, 71.528052)
  arc A75 (64.095126, 70.511318) -> (60.233181, 71.528052) centre (60.449397, 64.50638) ccw
  line L27 (64.095126, 70.511318) -> (153.154364, 16.44151)
  arc A76 (154.18878, 0.023621) -> (153.154364, 16.44151) centre (147.951739, 7.872185) ccw
  line L28 (154.18878, 0.023621) -> (141.440781, -10.106867)
  arc A77 (131.660668, -10.24148) -> (141.440781, -10.106867) centre (136.463592, -3.843674) ccw
  line L29 (131.660668, -10.24148) -> (40.231602, 58.395617)
  arc A78 (37.546552, 65.319255) -> (40.231602, 58.395617) centre (44.44917, 64.013691) ccw
  line L30 (37.546552, 65.319255) -> (62.581181, 46.525404)
  arc A79 (62.581181, 46.525404) -> (66.303447, 51.483704) centre (64.442314, 49.004554) ccw
  line L31 (66.303447, 51.483704) -> (41.268818, 70.277554)
  arc A80 (44.232954, 71.035362) -> (41.268818, 70.277554) centre (44.44917, 64.013691) ccw
  line L32 (44.232954, 71.035362) -> (46.496021, 71.105048)
  line L33 (46.496021, 71.105048) -> (58.588264, 62.02723)
  arc A81 (58.588264, 62.02723) -> (62.310529, 66.98553) centre (60.449397, 64.50638) ccw
  point P0 (0, 0)